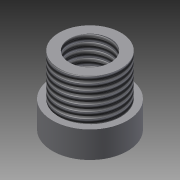
# Autodesk Inventor part: AcmeRoundNut
Saved by Autodesk Inventor 2013 (Build 170138000, 138)
## iProperties
Created: 2012-12-07
Part Number: AcmeRoundNut
Material: Generic
Document SubType Name: Modeling
Designer: istvan.burbank
Density: 1 g/cm^3
Author: istvan.burbank
Autodesk Inventor part; units mm, degrees
ref_plane "YZ Plane" through (0, 0, 0) normal (1, 0, 0) x (0, 1, 0)
ref_plane "XZ Plane" through (0, 0, 0) normal (0, 1, 0) x (-1, 0, 0)
ref_plane "XY Plane" through (0, 0, 0) normal (0, 0, 1) x (1, 0, 0)
sketch "Sketch1" plane through (0, 0, 0) normal (0, 1, 0) x (-1, 0, 0)
  circle A0 centre (0, 0) radius 4.7625
  circle A1 centre (0, 0) radius 8.636
  dimension "d0" = 9.525
  dimension "d1" = 17.272
  constraints: 2 centre point, 2 coincident
  measures "d0" diameter of A0
  measures "d1" diameter of A1
extrude "Extrusion1" add sketch "Sketch1" along normal blind 15.748
thread "Thread1" size "3/8-16 UNC" class "2B" standard "ANSI Unified Screw Threads" length 15.2654
sketch "Sketch2" plane through (0, 15.748, 0) normal (0, 1, 0) x (1, 0, 0)
  circle A0 centre (0, 0) radius 8.636 projected
  circle A1 centre (0, 0) radius 7.1374
  dimension "d6" = 14.2748
  constraints: 1 centre point, 1 coincident
  measures "d6" diameter of A1
extrude "Extrusion2" cut sketch "Sketch2" against normal blind 9.652
thread "Thread2" size "9/16-18 UNF" class "2A" standard "ANSI Unified Screw Threads" length 25.4
body "Solid1"
